Autodesk Inventor part; units mm, degrees
(part 3 of 16)
  spline S11 degree 3 poles (-7.8004, 116.1965) (-7.729, 116.082) (-7.6593, 115.9666) (-7.5915, 115.85) (-7.5548, 115.787) (-7.5187, 115.7236) (-7.4832, 115.66) (-7.4495, 115.5997) (-7.4164, 115.5392) (-7.3838, 115.4783) (-7.3531, 115.4209) (-7.3228, 115.3632) (-7.2931, 115.3052) (-7.2652, 115.2507) (-7.2377, 115.196) (-7.2107, 115.141) (-7.1855, 115.0895) (-7.1607, 115.0378) (-7.1363, 114.9858) (-7.1136, 114.9374) (-7.0914, 114.8888) (-7.0695, 114.8399) (-7.0493, 114.7947) (-7.0295, 114.7492) (-7.01, 114.7036) (-6.9921, 114.6615) (-6.9746, 114.6193) (-6.9574, 114.577) (-6.9417, 114.5382) (-6.9264, 114.4993) (-6.9114, 114.4603) (-6.8977, 114.4249) (-6.8844, 114.3893) (-6.8714, 114.3537) (-6.8598, 114.3217) (-6.8484, 114.2896) (-6.8373, 114.2574) (-6.8227, 114.2149) (-6.8087, 114.1721) (-6.7951, 114.1292) (-6.792, 114.1196) (-6.789, 114.11) (-6.7858, 114.1005) (-6.7828, 114.0911) (-6.7796, 114.0818) (-6.7764, 114.0725) (-6.7732, 114.0634) (-6.7699, 114.0544) (-6.7666, 114.0453) (-6.7633, 114.0365) (-6.76, 114.0277) (-6.7566, 114.0189) (-6.7532, 114.0102) (-6.7497, 114.0016) (-6.7462, 113.9931) (-6.7427, 113.9847) (-6.7391, 113.9763) (-6.7355, 113.9679) (-6.7318, 113.9597) (-6.7281, 113.9515) (-6.7243, 113.9433) (-6.7205, 113.9352) (-6.7166, 113.9272) (-6.7127, 113.9192) (-6.7087, 113.9113) (-6.7046, 113.9034) (-6.7004, 113.8955) (-6.6962, 113.8877) (-6.6919, 113.8799) (-6.6875, 113.8722) (-6.683, 113.8644) (-6.6784, 113.8566) (-6.6737, 113.849) (-6.6689, 113.8412) (-6.6639, 113.8335) (-6.6588, 113.8259) (-6.6536, 113.8181) (-6.6482, 113.8104) (-6.6426, 113.8028) (-6.6368, 113.7949) (-6.6309, 113.7871) (-6.6247, 113.7795) (-6.6182, 113.7715) (-6.6115, 113.7636) (-6.6046, 113.7559) (-6.5972, 113.7476) (-6.5896, 113.7396) (-6.5817, 113.7318) (-6.5731, 113.7234) (-6.5643, 113.7152) (-6.5551, 113.7074) (-6.5451, 113.6988) (-6.5346, 113.6906) (-6.5239, 113.6828) (-6.5119, 113.6741) (-6.4995, 113.666) (-6.4867, 113.6585) (-6.4723, 113.65) (-6.4575, 113.6424) (-6.4423, 113.6356) (-6.4252, 113.628) (-6.4076, 113.6214) (-6.3897, 113.6161) (-6.3697, 113.6101) (-6.3494, 113.6056) (-6.3288, 113.6026) (-6.3064, 113.5994) (-6.2838, 113.5978) (-6.2613, 113.5983) (-6.2398, 113.5988) (-6.2183, 113.6012) (-6.1969, 113.6039) (-6.0912, 113.6175) (-5.987, 113.6399) (-5.8819, 113.6571) (-5.7768, 113.6744) (-5.6709, 113.6865) (-5.5664, 113.7076) (-5.5453, 113.7118) (-5.5242, 113.7165) (-5.5036, 113.7229) (-5.4821, 113.7296) (-5.4612, 113.7383) (-5.4411, 113.7486) (-5.4225, 113.758) (-5.4047, 113.7688) (-5.3877, 113.7808) (-5.3724, 113.7916) (-5.3579, 113.8034) (-5.3441, 113.8161) (-5.3319, 113.8274) (-5.3203, 113.8394) (-5.3094, 113.852) (-5.2997, 113.8632) (-5.2905, 113.8749) (-5.2819, 113.887) (-5.2742, 113.8978) (-5.267, 113.9089) (-5.2602, 113.9203) (-5.254, 113.9307) (-5.2483, 113.9412) (-5.2428, 113.952) (-5.2379, 113.9619) (-5.2332, 113.9719) (-5.2288, 113.9821) (-5.2247, 113.9916) (-5.2209, 114.0012) (-5.2174, 114.0109) (-5.214, 114.0201) (-5.2108, 114.0293) (-5.2078, 114.0387) (-5.205, 114.0477) (-5.2024, 114.0567) (-5.1999, 114.0658) (-5.1975, 114.0746) (-5.1953, 114.0835) (-5.1932, 114.0924) (-5.1912, 114.1012) (-5.1893, 114.1099) (-5.1875, 114.1188) (-5.1858, 114.1275) (-5.1842, 114.1363) (-5.1828, 114.145) (-5.1813, 114.1538) (-5.18, 114.1626) (-5.1788, 114.1714) (-5.1776, 114.1802) (-5.1765, 114.1891) (-5.1755, 114.198) (-5.1745, 114.2069) (-5.1736, 114.2159) (-5.1728, 114.2248) (-5.172, 114.2339) (-5.1713, 114.243) (-5.1707, 114.2521) (-5.17, 114.2614) (-5.1695, 114.2706) (-5.1691, 114.2799) (-5.1687, 114.2893) (-5.1683, 114.2987) (-5.168, 114.3082) (-5.1678, 114.3178) (-5.1676, 114.3274) (-5.1675, 114.337) (-5.1674, 114.3469) (-5.1674, 114.3567) (-5.1675, 114.3666) (-5.1676, 114.3766) (-5.1678, 114.3867) (-5.1679, 114.3967) (-5.1687, 114.4417) (-5.1692, 114.4867) (-5.1689, 114.5317) (-5.1688, 114.5658) (-5.1682, 114.5998) (-5.1674, 114.6339) (-5.1666, 114.6718) (-5.1653, 114.7097) (-5.1638, 114.7476) (-5.162, 114.7894) (-5.1599, 114.8311) (-5.1575, 114.8729) (-5.1548, 114.9185) (-5.1517, 114.9641) (-5.1482, 115.0097) (-5.1444, 115.0591) (-5.1401, 115.1085) (-5.1354, 115.1579) (-5.1304, 115.2112) (-5.1249, 115.2643) (-5.1189, 115.3175) (-5.1125, 115.3745) (-5.1055, 115.4314) (-5.0981, 115.4883) (-5.0901, 115.549) (-5.0816, 115.6097) (-5.0726, 115.6703) (-5.063, 115.7347) (-5.0528, 115.7991) (-5.0421, 115.8633) (-5.0307, 115.9314) (-5.0187, 115.9994) (-5.0061, 116.0672) (-4.9929, 116.1389) (-4.9789, 116.2105) (-4.9643, 116.2819) (-4.9374, 116.4141) (-4.9084, 116.5458) (-4.8774, 116.677) knots 0 0 0 0 0.057795 0.057795 0.057795 0.089038 0.089038 0.089038 0.118617 0.118617 0.118617 0.14653 0.14653 0.14653 0.172778 0.172778 0.172778 0.19736 0.19736 0.19736 0.220277 0.220277 0.220277 0.241529 0.241529 0.241529 0.261115 0.261115 0.261115 0.279036 0.279036 0.279036 0.295292 0.295292 0.295292 0.309882 0.309882 0.309882 0.329164 0.329164 0.329164 0.333477 0.333477 0.333477 0.337694 0.337694 0.337694 0.34182 0.34182 0.34182 0.345864 0.345864 0.345864 0.349834 0.349834 0.349834 0.353742 0.353742 0.353742 0.3576 0.3576 0.3576 0.361424 0.361424 0.361424 0.365232 0.365232 0.365232 0.369048 0.369048 0.369048 0.372899 0.372899 0.372899 0.376819 0.376819 0.376819 0.380853 0.380853 0.380853 0.385052 0.385052 0.385052 0.389482 0.389482 0.389482 0.394225 0.394225 0.394225 0.399381 0.399381 0.399381 0.405067 0.405067 0.405067 0.411413 0.411413 0.411413 0.418548 0.418548 0.418548 0.426565 0.426565 0.426565 0.435472 0.435472 0.435472 0.445133 0.445133 0.445133 0.45436 0.45436 0.45436 0.5 0.5 0.5 0.54564 0.54564 0.54564 0.554867 0.554867 0.554867 0.564528 0.564528 0.564528 0.573435 0.573435 0.573435 0.581452 0.581452 0.581452 0.588587 0.588587 0.588587 0.594933 0.594933 0.594933 0.600619 0.600619 0.600619 0.605775 0.605775 0.605775 0.610518 0.610518 0.610518 0.614948 0.614948 0.614948 0.619147 0.619147 0.619147 0.623181 0.623181 0.623181 0.627101 0.627101 0.627101 0.630952 0.630952 0.630952 0.634768 0.634768 0.634768 0.638576 0.638576 0.638576 0.6424 0.6424 0.6424 0.646258 0.646258 0.646258 0.650166 0.650166 0.650166 0.654136 0.654136 0.654136 0.65818 0.65818 0.65818 0.662306 0.662306 0.662306 0.666523 0.666523 0.666523 0.670836 0.670836 0.670836 0.690118 0.690118 0.690118 0.704708 0.704708 0.704708 0.720964 0.720964 0.720964 0.738885 0.738885 0.738885 0.758471 0.758471 0.758471 0.779723 0.779723 0.779723 0.80264 0.80264 0.80264 0.827222 0.827222 0.827222 0.85347 0.85347 0.85347 0.881383 0.881383 0.881383 0.910962 0.910962 0.910962 0.942205 0.942205 0.942205 1 1 1 1
  arc A213 (-7.8004, 116.1965) -> (-8.9334, 115.9487) centre (0.0435, 77.6158) ccw
  spline S12 degree 3 poles (-11.7902, 115.1652) (-11.7073, 115.0589) (-11.6259, 114.9513) (-11.5462, 114.8425) (-11.5032, 114.7836) (-11.4606, 114.7244) (-11.4186, 114.6648) (-11.3789, 114.6084) (-11.3396, 114.5516) (-11.3008, 114.4945) (-11.2643, 114.4406) (-11.2282, 114.3864) (-11.1925, 114.3319) (-11.1591, 114.2806) (-11.126, 114.229) (-11.0934, 114.1771) (-11.0629, 114.1286) (-11.0329, 114.0797) (-11.0032, 114.0306) (-10.9756, 113.9848) (-10.9484, 113.9388) (-10.9216, 113.8925) (-10.8967, 113.8496) (-10.8722, 113.8065) (-10.8481, 113.7631) (-10.8259, 113.7232) (-10.8041, 113.683) (-10.7826, 113.6427) (-10.7629, 113.6058) (-10.7436, 113.5687) (-10.7246, 113.5315) (-10.7073, 113.4977) (-10.6904, 113.4637) (-10.6737, 113.4296) (-10.6588, 113.399) (-10.6441, 113.3683) (-10.6297, 113.3375) (-10.6108, 113.2967) (-10.5924, 113.2556) (-10.5743, 113.2144) (-10.5703, 113.2052) (-10.5662, 113.1959) (-10.5621, 113.1868) (-10.5581, 113.1778) (-10.554, 113.1689) (-10.5498, 113.16) (-10.5457, 113.1512) (-10.5415, 113.1426) (-10.5372, 113.1339) (-10.5331, 113.1255) (-10.5288, 113.117) (-10.5245, 113.1087) (-10.5202, 113.1004) (-10.5159, 113.0922) (-10.5115, 113.0841) (-10.5071, 113.0761) (-10.5027, 113.0681) (-10.4982, 113.0602) (-10.4937, 113.0524) (-10.4891, 113.0446) (-10.4845, 113.0369) (-10.4799, 113.0293) (-10.4752, 113.0217) (-10.4704, 113.0141) (-10.4656, 113.0066) (-10.4607, 112.9992) (-10.4558, 112.9919) (-10.4508, 112.9845) (-10.4457, 112.9772) (-10.4404, 112.97) (-10.4352, 112.9627) (-10.4298, 112.9555) (-10.4243, 112.9484) (-10.4187, 112.9411) (-10.413, 112.934) (-10.4071, 112.927) (-10.4011, 112.9198) (-10.3949, 112.9126) (-10.3886, 112.9057) (-10.382, 112.8984) (-10.3752, 112.8913) (-10.3683, 112.8844) (-10.361, 112.877) (-10.3535, 112.8699) (-10.3459, 112.863) (-10.3377, 112.8556) (-10.3292, 112.8484) (-10.3206, 112.8415) (-10.3112, 112.834) (-10.3015, 112.8268) (-10.2916, 112.82) (-10.2807, 112.8124) (-10.2694, 112.8053) (-10.2579, 112.7987) (-10.2451, 112.7913) (-10.2319, 112.7845) (-10.2184, 112.7784) (-10.2032, 112.7715) (-10.1877, 112.7655) (-10.1719, 112.7603) (-10.1541, 112.7545) (-10.1359, 112.7499) (-10.1175, 112.7464) (-10.097, 112.7426) (-10.0763, 112.7402) (-10.0555, 112.7394) (-10.033, 112.7385) (-10.0103, 112.7393) (-9.988, 112.7422) (-9.9666, 112.7449) (-9.9455, 112.7495) (-9.9245, 112.7545) (-9.8208, 112.779) (-9.7195, 112.8122) (-9.6168, 112.8403) (-9.5141, 112.8685) (-9.41, 112.8916) (-9.3083, 112.9235) (-9.2877, 112.9299) (-9.2672, 112.9367) (-9.2475, 112.9453) (-9.2268, 112.9542) (-9.2069, 112.965) (-9.1879, 112.9773) (-9.1705, 112.9887) (-9.1539, 113.0012) (-9.1382, 113.015) (-9.1242, 113.0273) (-9.1109, 113.0406) (-9.0986, 113.0547) (-9.0876, 113.0672) (-9.0773, 113.0803) (-9.0678, 113.094) (-9.0593, 113.1061) (-9.0514, 113.1187) (-9.0441, 113.1316) (-9.0376, 113.1432) (-9.0316, 113.155) (-9.026, 113.167) (-9.021, 113.178) (-9.0163, 113.1891) (-9.0121, 113.2003) (-9.0081, 113.2107) (-9.0045, 113.2212) (-9.0013, 113.2317) (-8.9982, 113.2416) (-8.9954, 113.2516) (-8.9929, 113.2616) (-8.9904, 113.2711) (-8.9883, 113.2806) (-8.9863, 113.2902) (-8.9844, 113.2995) (-8.9827, 113.3087) (-8.9812, 113.318) (-8.9798, 113.3271) (-8.9785, 113.3361) (-8.9774, 113.3452) (-8.9763, 113.3541) (-8.9753, 113.3631) (-8.9745, 113.372) (-8.9737, 113.3809) (-8.973, 113.3898) (-8.9725, 113.3986) (-8.972, 113.4075) (-8.9716, 113.4164) (-8.9713, 113.4253) (-8.971, 113.4342) (-8.9708, 113.4431) (-8.9708, 113.452) (-8.9707, 113.461) (-8.9707, 113.47) (-8.9709, 113.479) (-8.971, 113.4882) (-8.9713, 113.4973) (-8.9716, 113.5064) (-8.972, 113.5156) (-8.9724, 113.5249) (-8.973, 113.5342) (-8.9735, 113.5436) (-8.9742, 113.553) (-8.9749, 113.5624) (-8.9756, 113.572) (-8.9765, 113.5816) (-8.9774, 113.5912) (-8.9783, 113.601) (-8.9793, 113.6108) (-8.9804, 113.6205) (-8.9816, 113.6305) (-8.9828, 113.6405) (-8.984, 113.6505) (-8.9895, 113.6952) (-8.9947, 113.7399) (-8.9992, 113.7846) (-9.0026, 113.8185) (-9.0056, 113.8524) (-9.0083, 113.8864) (-9.0114, 113.9242) (-9.0142, 113.962) (-9.0166, 113.9999) (-9.0192, 114.0416) (-9.0215, 114.0834) (-9.0234, 114.1251) (-9.0255, 114.1708) (-9.0272, 114.2165) (-9.0285, 114.2622) (-9.0299, 114.3117) (-9.0308, 114.3613) (-9.0313, 114.4109) (-9.0318, 114.4644) (-9.0319, 114.5179) (-9.0315, 114.5713) (-9.0311, 114.6287) (-9.0301, 114.6861) (-9.0287, 114.7434) (-9.0271, 114.8046) (-9.025, 114.8659) (-9.0224, 114.927) (-9.0196, 114.9921) (-9.0162, 115.0572) (-9.0122, 115.1222) (-9.008, 115.1911) (-9.0032, 115.2599) (-8.9978, 115.3287) (-8.992, 115.4014) (-8.9856, 115.4741) (-8.9786, 115.5466) (-8.9656, 115.6809) (-8.9505, 115.8149) (-8.9334, 115.9487) knots 0 0 0 0 0.057795 0.057795 0.057795 0.089038 0.089038 0.089038 0.118617 0.118617 0.118617 0.14653 0.14653 0.14653 0.172778 0.172778 0.172778 0.19736 0.19736 0.19736 0.220277 0.220277 0.220277 0.241529 0.241529 0.241529 0.261115 0.261115 0.261115 0.279036 0.279036 0.279036 0.295292 0.295292 0.295292 0.309882 0.309882 0.309882 0.329164 0.329164 0.329164 0.333477 0.333477 0.333477 0.337694 0.337694 0.337694 0.34182 0.34182 0.34182 0.345864 0.345864 0.345864 0.349834 0.349834 0.349834 0.353742 0.353742 0.353742 0.3576 0.3576 0.3576 0.361424 0.361424 0.361424 0.365232 0.365232 0.365232 0.369048 0.369048 0.369048 0.372899 0.372899 0.372899 0.376819 0.376819 0.376819 0.380853 0.380853 0.380853 0.385052 0.385052 0.385052 0.389482 0.389482 0.389482 0.394225 0.394225 0.394225 0.399381 0.399381 0.399381 0.405067 0.405067 0.405067 0.411413 0.411413 0.411413 0.418548 0.418548 0.418548 0.426565 0.426565 0.426565 0.435472 0.435472 0.435472 0.445133 0.445133 0.445133 0.45436 0.45436 0.45436 0.5 0.5 0.5 0.54564 0.54564 0.54564 0.554867 0.554867 0.554867 0.564528 0.564528 0.564528 0.573435 0.573435 0.573435 0.581452 0.581452 0.581452 0.588587 0.588587 0.588587 0.594933 0.594933 0.594933 0.600619 0.600619 0.600619 0.605775 0.605775 0.605775 0.610518 0.610518 0.610518 0.614948 0.614948 0.614948 0.619147 0.619147 0.619147 0.623181 0.623181 0.623181 0.627101 0.627101 0.627101 0.630952 0.630952 0.630952 0.634768 0.634768 0.634768 0.638576 0.638576 0.638576 0.6424 0.6424 0.6424 0.646258 0.646258 0.646258 0.650166 0.650166 0.650166 0.654136 0.654136 0.654136 0.65818 0.65818 0.65818 0.662306 0.662306 0.662306 0.666523 0.666523 0.666523 0.670836 0.670836 0.670836 0.690118 0.690118 0.690118 0.704708 0.704708 0.704708 0.720964 0.720964 0.720964 0.738885 0.738885 0.738885 0.758471 0.758471 0.758471 0.779723 0.779723 0.779723 0.80264 0.80264 0.80264 0.827222 0.827222 0.827222 0.85347 0.85347 0.85347 0.881383 0.881383 0.881383 0.910962 0.910962 0.910962 0.942205 0.942205 0.942205 1 1 1 1
  arc A214 (-11.7902, 115.1652) -> (-12.8911, 114.8003) centre (0.0435, 77.6158) ccw
  spline S13 degree 3 poles (-15.6504, 113.7226) (-15.5568, 113.6255) (-15.4646, 113.527) (-15.374, 113.4271) (-15.325, 113.3731) (-15.2765, 113.3186) (-15.2285, 113.2638) (-15.1831, 113.2118) (-15.1381, 113.1595) (-15.0936, 113.1067) (-15.0516, 113.0569) (-15.01, 113.0068) (-14.9689, 112.9563) (-14.9302, 112.9088) (-14.892, 112.8609) (-14.8541, 112.8127) (-14.8187, 112.7676) (-14.7837, 112.7222) (-14.7491, 112.6764) (-14.7168, 112.6338) (-14.6849, 112.5908) (-14.6535, 112.5476) (-14.6242, 112.5075) (-14.5954, 112.4672) (-14.5669, 112.4266) (-14.5406, 112.3892) (-14.5147, 112.3516) (-14.4891, 112.3137) (-14.4657, 112.2791) (-14.4426, 112.2442) (-14.4198, 112.2091) (-14.3991, 112.1773) (-14.3787, 112.1454) (-14.3586, 112.1132) (-14.3405, 112.0843) (-14.3227, 112.0553) (-14.3052, 112.0261) (-14.2821, 111.9875) (-14.2595, 111.9486) (-14.2372, 111.9095) (-14.2322, 111.9008) (-14.2273, 111.892) (-14.2222, 111.8833) (-14.2173, 111.8748) (-14.2122, 111.8664) (-14.2071, 111.8579) (-14.2021, 111.8497) (-14.1971, 111.8415) (-14.1919, 111.8334) (-14.1869, 111.8254) (-14.1818, 111.8175) (-14.1766, 111.8096) (-14.1715, 111.8018) (-14.1663, 111.7941) (-14.1611, 111.7865) (-14.1559, 111.779) (-14.1507, 111.7715) (-14.1454, 111.7641) (-14.1401, 111.7568) (-14.1348, 111.7496) (-14.1293, 111.7424) (-14.124, 111.7353) (-14.1185, 111.7282) (-14.1129, 111.7212) (-14.1074, 111.7143) (-14.1018, 111.7074) (-14.096, 111.7006) (-14.0903, 111.6938) (-14.0845, 111.6871) (-14.0785, 111.6804) (-14.0725, 111.6737) (-14.0664, 111.6671) (-14.0602, 111.6606) (-14.0539, 111.654) (-14.0475, 111.6475) (-14.0409, 111.6412) (-14.0341, 111.6346) (-14.0273, 111.6282) (-14.0202, 111.6219) (-14.0129, 111.6154) (-14.0055, 111.609) (-13.9979, 111.6028) (-13.9898, 111.5963) (-13.9817, 111.59) (-13.9733, 111.5839) (-13.9643, 111.5774) (-13.9552, 111.5711) (-13.9459, 111.5652) (-13.9357, 111.5587) (-13.9254, 111.5526) (-13.9148, 111.5468) (-13.9032, 111.5404) (-13.8913, 111.5346) (-13.8791, 111.5292) (-13.8656, 111.5232) (-13.8517, 111.5178) (-13.8377, 111.5131) (-13.8219, 111.5079) (-13.8058, 111.5035) (-13.7895, 111.5) (-13.7712, 111.4961) (-13.7526, 111.4934) (-13.734, 111.4918) (-13.7132, 111.4902) (-13.6924, 111.49) (-13.6716, 111.4914) (-13.6491, 111.4928) (-13.6266, 111.496) (-13.6047, 111.5012) (-13.5838, 111.5061) (-13.5633, 111.5129) (-13.5429, 111.52) (-13.4423, 111.5553) (-13.345, 111.5989) (-13.2458, 111.6376) (-13.1467, 111.6763) (-13.0456, 111.7102) (-12.9477, 111.7525) (-12.9279, 111.7611) (-12.9083, 111.77) (-12.8895, 111.7805) (-12.8699, 111.7916) (-12.8512, 111.8045) (-12.8337, 111.8187) (-12.8175, 111.8318) (-12.8023, 111.846) (-12.7882, 111.8613) (-12.7755, 111.8751) (-12.7637, 111.8897) (-12.7529, 111.9049) (-12.7432, 111.9185) (-12.7344, 111.9327) (-12.7263, 111.9473) (-12.7192, 111.9602) (-12.7126, 111.9735) (-12.7067, 111.9871) (-12.7015, 111.9993) (-12.6967, 112.0117) (-12.6924, 112.0243) (-12.6886, 112.0357) (-12.6851, 112.0472) (-12.682, 112.0588) (-12.6792, 112.0695) (-12.6768, 112.0803) (-12.6746, 112.0912) (-12.6726, 112.1013) (-12.6708, 112.1115) (-12.6694, 112.1218) (-12.668, 112.1315) (-12.6668, 112.1412) (-12.6658, 112.1509) (-12.6649, 112.1603) (-12.6642, 112.1697) (-12.6637, 112.1791) (-12.6632, 112.1882) (-12.6629, 112.1974) (-12.6627, 112.2065) (-12.6625, 112.2155) (-12.6625, 112.2245) (-12.6626, 112.2335) (-12.6628, 112.2424) (-12.663, 112.2513) (-12.6634, 112.2602) (-12.6638, 112.2691) (-12.6644, 112.2779) (-12.665, 112.2868) (-12.6656, 112.2957) (-12.6664, 112.3046) (-12.6673, 112.3135) (-12.6682, 112.3224) (-12.6691, 112.3314) (-12.6702, 112.3403) (-12.6713, 112.3494) (-12.6725, 112.3584) (-12.6738, 112.3674) (-12.6752, 112.3766) (-12.6766, 112.3858) (-12.6781, 112.3949) (-12.6796, 112.4042) (-12.6812, 112.4135) (-12.6829, 112.4228) (-12.6847, 112.4323) (-12.6865, 112.4417) (-12.6884, 112.4512) (-12.6904, 112.4608) (-12.6924, 112.4704) (-12.6945, 112.48) (-12.6967, 112.4899) (-12.699, 112.4997) (-12.7012, 112.5095) (-12.7114, 112.5533) (-12.7211, 112.5972) (-12.7303, 112.6413) (-12.7372, 112.6746) (-12.7438, 112.708) (-12.7501, 112.7415) (-12.7571, 112.7788) (-12.7638, 112.8161) (-12.7701, 112.8535) (-12.7771, 112.8947) (-12.7837, 112.936) (-12.79, 112.9774) (-12.7969, 113.0226) (-12.8033, 113.0678) (-12.8094, 113.1131) (-12.8159, 113.1623) (-12.822, 113.2115) (-12.8277, 113.2608) (-12.8339, 113.3139) (-12.8395, 113.3671) (-12.8447, 113.4203) (-12.8503, 113.4774) (-12.8553, 113.5345) (-12.8599, 113.5917) (-12.8647, 113.6528) (-12.869, 113.7139) (-12.8728, 113.775) (-12.8768, 113.84) (-12.8802, 113.9051) (-12.8831, 113.9701) (-12.8861, 114.0391) (-12.8885, 114.1081) (-12.8903, 114.1771) (-12.8922, 114.25) (-12.8934, 114.3229) (-12.8941, 114.3958) (-12.8952, 114.5306) (-12.8941, 114.6655) (-12.8911, 114.8003) knots 0 0 0 0 0.057795 0.057795 0.057795 0.089038 0.089038 0.089038 0.118617 0.118617 0.118617 0.14653 0.14653 0.14653 0.172778 0.172778 0.172778 0.19736 0.19736 0.19736 0.220277 0.220277 0.220277 0.241529 0.241529 0.241529 0.261115 0.261115 0.261115 0.279036 0.279036 0.279036 0.295292 0.295292 0.295292 0.309882 0.309882 0.309882 0.329164 0.329164 0.329164 0.333477 0.333477 0.333477 0.337694 0.337694 0.337694 0.34182 0.34182 0.34182 0.345864 0.345864 0.345864 0.349834 0.349834 0.349834 0.353742 0.353742 0.353742 0.3576 0.3576 0.3576 0.361424 0.361424 0.361424 0.365232 0.365232 0.365232 0.369048 0.369048 0.369048 0.372899 0.372899 0.372899 0.376819 0.376819 0.376819 0.380853 0.380853 0.380853 0.385052 0.385052 0.385052 0.389482 0.389482 0.389482 0.394225 0.394225 0.394225 0.399381 0.399381 0.399381 0.405067 0.405067 0.405067 0.411413 0.411413 0.411413 0.418548 0.418548 0.418548 0.426565 0.426565 0.426565 0.435472 0.435472 0.435472 0.445133 0.445133 0.445133 0.45436 0.45436 0.45436 0.5 0.5 0.5 0.54564 0.54564 0.54564 0.554867 0.554867 0.554867 0.564528 0.564528 0.564528 0.573435 0.573435 0.573435 0.581452 0.581452 0.581452 0.588587 0.588587 0.588587 0.594933 0.594933 0.594933 0.600619 0.600619 0.600619 0.605775 0.605775 0.605775 0.610518 0.610518 0.610518 0.614948 0.614948 0.614948 0.619147 0.619147 0.619147 0.623181 0.623181 0.623181 0.627101 0.627101 0.627101 0.630952 0.630952 0.630952 0.634768 0.634768 0.634768 0.638576 0.638576 0.638576 0.6424 0.6424 0.6424 0.646258 0.646258 0.646258 0.650166 0.650166 0.650166 0.654136 0.654136 0.654136 0.65818 0.65818 0.65818 0.662306 0.662306 0.662306 0.666523 0.666523 0.666523 0.670836 0.670836 0.670836 0.690118 0.690118 0.690118 0.704708 0.704708 0.704708 0.720964 0.720964 0.720964 0.738885 0.738885 0.738885 0.758471 0.758471 0.758471 0.779723 0.779723 0.779723 0.80264 0.80264 0.80264 0.827222 0.827222 0.827222 0.85347 0.85347 0.85347 0.881383 0.881383 0.881383 0.910962 0.910962 0.910962 0.942205 0.942205 0.942205 1 1 1 1
  arc A215 (-15.6504, 113.7226) -> (-16.7071, 113.2446) centre (0.0435, 77.6158) ccw
  spline S14 degree 3 poles (-19.3386, 111.8843) (-19.2353, 111.7975) (-19.1334, 111.7092) (-19.0328, 111.6193) (-18.9785, 111.5707) (-18.9246, 111.5217) (-18.8711, 111.4721) (-18.8205, 111.4252) (-18.7702, 111.3778) (-18.7205, 111.33) (-18.6735, 111.2849) (-18.6269, 111.2394) (-18.5807, 111.1934) (-18.5373, 111.1502) (-18.4943, 111.1067) (-18.4516, 111.0627) (-18.4117, 111.0215) (-18.3721, 110.98) (-18.3329, 110.9381) (-18.2964, 110.8991) (-18.2602, 110.8597) (-18.2243, 110.82) (-18.1911, 110.7832) (-18.1582, 110.7461) (-18.1256, 110.7087) (-18.0955, 110.6743) (-18.0658, 110.6395) (-18.0364, 110.6046) (-18.0095, 110.5725) (-17.9829, 110.5403) (-17.9565, 110.5078) (-17.9326, 110.4783) (-17.909, 110.4487) (-17.8857, 110.4188) (-17.8647, 110.392) (-17.8439, 110.365) (-17.8235, 110.3378) (-17.7964, 110.3018) (-17.7699, 110.2655) (-17.7437, 110.2289) (-17.7378, 110.2207) (-17.7319, 110.2125) (-17.726, 110.2044) (-17.7202, 110.1965) (-17.7143, 110.1886) (-17.7083, 110.1808) (-17.7025, 110.1731) (-17.6966, 110.1655) (-17.6907, 110.1579) (-17.6848, 110.1505) (-17.6789, 110.1431) (-17.6729, 110.1358) (-17.667, 110.1287) (-17.6611, 110.1216) (-17.6551, 110.1145) (-17.6492, 110.1076) (-17.6432, 110.1007) (-17.6371, 110.0939) (-17.6311, 110.0872) (-17.625, 110.0805) (-17.6189, 110.074) (-17.6128, 110.0674) (-17.6066, 110.061) (-17.6004, 110.0546) (-17.5941, 110.0483) (-17.5878, 110.0421) (-17.5814, 110.0359) (-17.575, 110.0297) (-17.5685, 110.0236) (-17.5619, 110.0177) (-17.5552, 110.0116) (-17.5485, 110.0057) (-17.5416, 109.9999) (-17.5346, 109.994) (-17.5276, 109.9882) (-17.5204, 109.9825) (-17.513, 109.9767) (-17.5054, 109.9711) (-17.4978, 109.9656) (-17.4898, 109.9598) (-17.4818, 109.9543) (-17.4736, 109.9489) (-17.4649, 109.9433) (-17.4561, 109.9379) (-17.4471, 109.9327) (-17.4376, 109.9271) (-17.4278, 109.9219) (-17.4179, 109.9169) (-17.4072, 109.9115) (-17.3962, 109.9065) (-17.3851, 109.9019) (-17.3729, 109.8968) (-17.3604, 109.8922) (-17.3478, 109.8881) (-17.3337, 109.8835) (-17.3194, 109.8797) (-17.3049, 109.8765) (-17.2886, 109.8729) (-17.2722, 109.8702) (-17.2556, 109.8684) (-17.237, 109.8665) (-17.2182, 109.8657) (-17.1995, 109.8661) (-17.1787, 109.8666) (-17.158, 109.8687) (-17.1375, 109.8722) (-17.1152, 109.876) (-17.0932, 109.8815) (-17.0719, 109.8889) (-17.0516, 109.896) (-17.032, 109.9049) (-17.0125, 109.9141) (-16.9161, 109.9597) (-16.8239, 110.0132) (-16.7293, 110.0621) (-16.6347, 110.111) (-16.5377, 110.1553) (-16.4448, 110.2076) (-16.426, 110.2182) (-16.4074, 110.2291) (-16.3899, 110.2415) (-16.3715, 110.2546) (-16.3543, 110.2693) (-16.3383, 110.2853) (-16.3236, 110.3) (-16.3099, 110.3158) (-16.2975, 110.3324) (-16.2863, 110.3474) (-16.2761, 110.3632) (-16.2669, 110.3795) (-16.2588, 110.394) (-16.2515, 110.409) (-16.245, 110.4244) (-16.2392, 110.438) (-16.2341, 110.4519) (-16.2297, 110.4661) (-16.2257, 110.4787) (-16.2223, 110.4916) (-16.2193, 110.5045) (-16.2167, 110.5162) (-16.2144, 110.5281) (-16.2126, 110.54) (-16.2109, 110.5509) (-16.2096, 110.5619) (-16.2086, 110.5729) (-16.2076, 110.5832) (-16.207, 110.5936) (-16.2066, 110.6039) (-16.2062, 110.6137) (-16.206, 110.6235) (-16.2061, 110.6333) (-16.2062, 110.6427) (-16.2065, 110.6521) (-16.2069, 110.6615) (-16.2074, 110.6706) (-16.208, 110.6798) (-16.2088, 110.6889) (-16.2096, 110.6978) (-16.2105, 110.7068) (-16.2116, 110.7157) (-16.2126, 110.7245) (-16.2138, 110.7334) (-16.2152, 110.7422) (-16.2165, 110.751) (-16.2179, 110.7597) (-16.2195, 110.7685) (-16.2211, 110.7773) (-16.2228, 110.786) (-16.2245, 110.7948) (-16.2264, 110.8036) (-16.2283, 110.8124) (-16.2303, 110.8212) (-16.2323, 110.83) (-16.2345, 110.8389) (-16.2367, 110.8477) (-16.239, 110.8567) (-16.2413, 110.8657) (-16.2438, 110.8746) (-16.2463, 110.8837) (-16.2489, 110.8928) (-16.2515, 110.9018) (-16.2543, 110.9111) (-16.2571, 110.9203) (-16.26, 110.9295) (-16.2629, 110.9389) (-16.2659, 110.9482) (-16.2691, 110.9576) (-16.2722, 110.9671) (-16.2755, 110.9766) (-16.2788, 110.9861) (-16.2935, 111.0287) (-16.3078, 111.0713) (-16.3215, 111.1142) (-16.3318, 111.1466) (-16.3419, 111.1792) (-16.3516, 111.2118) (-16.3625, 111.2481) (-16.373, 111.2846) (-16.3833, 111.3211) (-16.3945, 111.3614) (-16.4054, 111.4017) (-16.416, 111.4422) (-16.4275, 111.4864) (-16.4387, 111.5308) (-16.4494, 111.5752) (-16.4611, 111.6234) (-16.4723, 111.6717) (-16.4831, 111.7201) (-16.4948, 111.7723) (-16.506, 111.8246) (-16.5167, 111.877) (-16.5282, 111.9332) (-16.5392, 111.9895) (-16.5497, 112.0459) (-16.5609, 112.1061) (-16.5716, 112.1664) (-16.5817, 112.2268) (-16.5925, 112.291) (-16.6027, 112.3554) (-16.6123, 112.4198) (-16.6226, 112.4881) (-16.6321, 112.5564) (-16.6412, 112.6248) (-16.6507, 112.6971) (-16.6595, 112.7695) (-16.6677, 112.8419) (-16.683, 112.976) (-16.696, 113.1102) (-16.7071, 113.2446) knots 0 0 0 0 0.057795 0.057795 0.057795 0.089038 0.089038 0.089038 0.118617 0.118617 0.118617 0.14653 0.14653 0.14653 0.172778 0.172778 0.172778 0.19736 0.19736 0.19736 0.220277 0.220277 0.220277 0.241529 0.241529 0.241529 0.261115 0.261115 0.261115 0.279036 0.279036 0.279036 0.295292 0.295292 0.295292 0.309882 0.309882 0.309882 0.329164 0.329164 0.329164 0.333477 0.333477 0.333477 0.337694 0.337694 0.337694 0.34182 0.34182 0.34182 0.345864 0.345864 0.345864 0.349834 0.349834 0.349834 0.353742 0.353742 0.353742 0.3576 0.3576 0.3576 0.361424 0.361424 0.361424 0.365232 0.365232 0.365232 0.369048 0.369048 0.369048 0.372899 0.372899 0.372899 0.376819 0.376819 0.376819 0.380853 0.380853 0.380853 0.385052 0.385052 0.385052 0.389482 0.389482 0.389482 0.394225 0.394225 0.394225 0.399381 0.399381 0.399381 0.405067 0.405067 0.405067 0.411413 0.411413 0.411413 0.418548 0.418548 0.418548 0.426565 0.426565 0.426565 0.435472 0.435472 0.435472 0.445133 0.445133 0.445133 0.45436 0.45436 0.45436 0.5 0.5 0.5 0.54564 0.54564 0.54564 0.554867 0.554867 0.554867 0.564528 0.564528 0.564528 0.573435 0.573435 0.573435 0.581452 0.581452 0.581452 0.588587 0.588587 0.588587 0.594933 0.594933 0.594933 0.600619 0.600619 0.600619 0.605775 0.605775 0.605775 0.610518 0.610518 0.610518 0.614948 0.614948 0.614948 0.619147 0.619147 0.619147 0.623181 0.623181 0.623181 0.627101 0.627101 0.627101 0.630952 0.630952 0.630952 0.634768 0.634768 0.634768 0.638576 0.638576 0.638576 0.6424 0.6424 0.6424 0.646258 0.646258 0.646258 0.650166 0.650166 0.650166 0.654136 0.654136 0.654136 0.65818 0.65818 0.65818 0.662306 0.662306 0.662306 0.666523 0.666523 0.666523 0.670836 0.670836 0.670836 0.690118 0.690118 0.690118 0.704708 0.704708 0.704708 0.720964 0.720964 0.720964 0.738885 0.738885 0.738885 0.758471 0.758471 0.758471 0.779723 0.779723 0.779723 0.80264 0.80264 0.80264 0.827222 0.827222 0.827222 0.85347 0.85347 0.85347 0.881383 0.881383 0.881383 0.910962 0.910962 0.910962 0.942205 0.942205 0.942205 1 1 1 1
  arc A216 (-19.3386, 111.8843) -> (-20.3396, 111.2985) centre (0.0435, 77.6158) ccw
  spline S15 degree 3 poles (-22.8144, 109.6706) (-22.7027, 109.5951) (-22.5921, 109.5179) (-22.4827, 109.439) (-22.4235, 109.3964) (-22.3648, 109.3532) (-22.3064, 109.3095) (-22.2512, 109.2682) (-22.1963, 109.2263) (-22.1418, 109.184) (-22.0903, 109.144) (-22.0392, 109.1036) (-21.9885, 109.0627) (-21.9408, 109.0243) (-21.8935, 108.9855) (-21.8465, 108.9462) (-21.8024, 108.9094) (-21.7587, 108.8723) (-21.7154, 108.8347) (-21.6749, 108.7997) (-21.6348, 108.7643) (-21.595, 108.7286) (-21.5581, 108.6955) (-21.5215, 108.662) (-21.4852, 108.6282) (-21.4517, 108.5971) (-21.4185, 108.5657) (-21.3856, 108.534) (-21.3555, 108.5049) (-21.3257, 108.4757) (-21.2961, 108.4461) (-21.2692, 108.4193) (-21.2426, 108.3923) (-21.2163, 108.365) (-21.1926, 108.3405) (-21.1692, 108.3158) (-21.146, 108.2909) (-21.1153, 108.258) (-21.0851, 108.2246) (-21.0552, 108.191) (-21.0485, 108.1835) (-21.0418, 108.1759) (-21.0351, 108.1685) (-21.0285, 108.1612) (-21.0218, 108.154) (-21.015, 108.1468) (-21.0085, 108.1398) (-21.0018, 108.1328) (-20.9951, 108.1259) (-20.9885, 108.1192) (-20.9819, 108.1125) (-20.9751, 108.1058) (-20.9686, 108.0993) (-20.9619, 108.0929) (-20.9552, 108.0865) (-20.9486, 108.0802) (-20.9419, 108.074) (-20.9351, 108.0679) (-20.9285, 108.0618) (-20.9217, 108.0558) (-20.9149, 108.0499) (-20.9082, 108.0441) (-20.9014, 108.0383) (-20.8945, 108.0327) (-20.8876, 108.027) (-20.8807, 108.0214) (-20.8737, 108.016) (-20.8667, 108.0105) (-20.8596, 108.0051) (-20.8524, 107.9999) (-20.8451, 107.9946) (-20.8378, 107.9894) (-20.8304, 107.9843) (-20.8228, 107.9792) (-20.8151, 107.9742) (-20.8074, 107.9693) (-20.7994, 107.9643) (-20.7913, 107.9595) (-20.7832, 107.9548) (-20.7747, 107.9499) (-20.7661, 107.9452) (-20.7573, 107.9408) (-20.7481, 107.9361) (-20.7388, 107.9316) (-20.7294, 107.9274) (-20.7193, 107.9229) (-20.709, 107.9186) (-20.6987, 107.9147) (-20.6874, 107.9105) (-20.676, 107.9067) (-20.6644, 107.9032) (-20.6517, 107.8994) (-20.6389, 107.8962) (-20.6259, 107.8934) (-20.6114, 107.8904) (-20.5967, 107.888) (-20.582, 107.8863) (-20.5655, 107.8845) (-20.5488, 107.8835) (-20.5321, 107.8835) (-20.5134, 107.8835) (-20.4947, 107.8847) (-20.4761, 107.8871) (-20.4555, 107.8898) (-20.4351, 107.8939) (-20.415, 107.8996) (-20.3933, 107.9057) (-20.372, 107.9134) (-20.3516, 107.9231) (-20.3322, 107.9323) (-20.3135, 107.9432) (-20.2951, 107.9544) (-20.204, 108.0098) (-20.1179, 108.0726) (-20.029, 108.1311) (-19.94, 108.1896) (-19.8482, 108.2438) (-19.7613, 108.3055) (-19.7437, 108.318) (-19.7263, 108.3308) (-19.7102, 108.345) (-19.6932, 108.3599) (-19.6777, 108.3764) (-19.6634, 108.3939) (-19.6503, 108.4101) (-19.6384, 108.4272) (-19.6278, 108.4451) (-19.6182, 108.4612) (-19.6097, 108.4779) (-19.6023, 108.4951) (-19.5958, 108.5104) (-19.59, 108.5261) (-19.5852, 108.542) (-19.5809, 108.5562) (-19.5773, 108.5706) (-19.5743, 108.5851) (-19.5717, 108.5981) (-19.5696, 108.6112) (-19.5681, 108.6244) (-19.5666, 108.6364) (-19.5657, 108.6484) (-19.5651, 108.6604) (-19.5646, 108.6714) (-19.5644, 108.6825) (-19.5645, 108.6936) (-19.5647, 108.7039) (-19.5651, 108.7143) (-19.5657, 108.7246) (-19.5664, 108.7344) (-19.5673, 108.7441) (-19.5684, 108.7539) (-19.5694, 108.7632) (-19.5707, 108.7725) (-19.5721, 108.7818) (-19.5735, 108.7909) (-19.5751, 108.7999) (-19.5768, 108.8089) (-19.5785, 108.8177) (-19.5804, 108.8265) (-19.5824, 108.8353) (-19.5844, 108.8439) (-19.5865, 108.8526) (-19.5887, 108.8612) (-19.591, 108.8698) (-19.5933, 108.8784) (-19.5958, 108.8869) (-19.5983, 108.8955) (-19.6009, 108.904) (-19.6036, 108.9125) (-19.6063, 108.9211) (-19.6091, 108.9297) (-19.612, 108.9382) (-19.615, 108.9468) (-19.6181, 108.9554) (-19.6212, 108.964) (-19.6244, 108.9726) (-19.6277, 108.9813) (-19.6311, 108.9899) (-19.6345, 108.9987) (-19.638, 109.0075) (-19.6416, 109.0162) (-19.6453, 109.0251) (-19.6491, 109.034) (-19.6529, 109.0428) (-19.6568, 109.0518) (-19.6608, 109.0608) (-19.6649, 109.0698) (-19.669, 109.0789) (-19.6733, 109.0881) (-19.6776, 109.0972) (-19.6966, 109.138) (-19.7153, 109.1789) (-19.7334, 109.2201) (-19.7471, 109.2513) (-19.7604, 109.2826) (-19.7735, 109.314) (-19.7882, 109.349) (-19.8024, 109.3841) (-19.8164, 109.4194) (-19.8319, 109.4583) (-19.8469, 109.4973) (-19.8617, 109.5364) (-19.8778, 109.5792) (-19.8935, 109.6221) (-19.9088, 109.6652) (-19.9254, 109.7119) (-19.9417, 109.7588) (-19.9575, 109.8058) (-19.9745, 109.8565) (-19.9911, 109.9073) (-20.0072, 109.9583) (-20.0246, 110.013) (-20.0414, 110.0678) (-20.0577, 110.1228) (-20.0752, 110.1815) (-20.0921, 110.2404) (-20.1085, 110.2994) (-20.1259, 110.3622) (-20.1428, 110.4251) (-20.1591, 110.4881) (-20.1764, 110.5549) (-20.1931, 110.6219) (-20.2092, 110.689) (-20.2262, 110.7599) (-20.2426, 110.831) (-20.2583, 110.9022) (-20.2875, 111.0339) (-20.3145, 111.166) (-20.3396, 111.2985) knots 0 0 0 0 0.057795 0.057795 0.057795 0.089038 0.089038 0.089038 0.118617 0.118617 0.118617 0.14653 0.14653 0.14653 0.172778 0.172778 0.172778 0.19736 0.19736 0.19736 0.220277 0.220277 0.220277 0.241529 0.241529 0.241529 0.261115 0.261115 0.261115 0.279036 0.279036 0.279036 0.295292 0.295292 0.295292 0.309882 0.309882 0.309882 0.329164 0.329164 0.329164 0.333477 0.333477 0.333477 0.337694 0.337694 0.337694 0.34182 0.34182 0.34182 0.345864 0.345864 0.345864 0.349834 0.349834 0.349834 0.353742 0.353742 0.353742 0.3576 0.3576 0.3576 0.361424 0.361424 0.361424 0.365232 0.365232 0.365232 0.369048 0.369048 0.369048 0.372899 0.372899 0.372899 0.376819 0.376819 0.376819 0.380853 0.380853 0.380853 0.385052 0.385052 0.385052 0.389482 0.389482 0.389482 0.394225 0.394225 0.394225 0.399381 0.399381 0.399381 0.405067 0.405067 0.405067 0.411413 0.411413 0.411413 0.418548 0.418548 0.418548 0.426565 0.426565 0.426565 0.435472 0.435472 0.435472 0.445133 0.445133 0.445133 0.45436 0.45436 0.45436 0.5 0.5 0.5 0.54564 0.54564 0.54564 0.554867 0.554867 0.554867 0.564528 0.564528 0.564528 0.573435 0.573435 0.573435 0.581452 0.581452 0.581452 0.588587 0.588587 0.588587 0.594933 0.594933 0.594933 0.600619 0.600619 0.600619 0.605775 0.605775 0.605775 0.610518 0.610518 0.610518 0.614948 0.614948 0.614948 0.619147 0.619147 0.619147 0.623181 0.623181 0.623181 0.627101 0.627101 0.627101 0.630952 0.630952 0.630952 0.634768 0.634768 0.634768 0.638576 0.638576 0.638576 0.6424 0.6424 0.6424 0.646258 0.646258 0.646258 0.650166 0.650166 0.650166 0.654136 0.654136 0.654136 0.65818 0.65818 0.65818 0.662306 0.662306 0.662306 0.666523 0.666523 0.666523 0.670836 0.670836 0.670836 0.690118 0.690118 0.690118 0.704708 0.704708 0.704708 0.720964 0.720964 0.720964 0.738885 0.738885 0.738885 0.758471 0.758471 0.758471 0.779723 0.779723 0.779723 0.80264 0.80264 0.80264 0.827222 0.827222 0.827222 0.85347 0.85347 0.85347 0.881383 0.881383 0.881383 0.910962 0.910962 0.910962 0.942205 0.942205 0.942205 1 1 1 1
  arc A217 (-22.8144, 109.6706) -> (-23.7487, 108.9834) centre (0.0435, 77.6158) ccw
  spline S16 degree 3 poles (-26.0399, 107.1057) (-25.9208, 107.0423) (-25.8027, 106.9771) (-25.6857, 106.9101) (-25.6224, 106.8738) (-25.5595, 106.8371) (-25.4969, 106.7997) (-25.4376, 106.7643) (-25.3786, 106.7285) (-25.32, 106.692) (-25.2647, 106.6577) (-25.2096, 106.6228) (-25.1549, 106.5875) (-25.1035, 106.5543) (-25.0523, 106.5206) (-25.0015, 106.4864) (-24.9538, 106.4545) (-24.9065, 106.4221) (-24.8594, 106.3893) (-24.8156, 106.3587) (-24.772, 106.3277) (-24.7287, 106.2963) (-24.6885, 106.2672) (-24.6486, 106.2378) (-24.6089, 106.208) (-24.5724, 106.1805) (-24.5361, 106.1528) (-24.5001, 106.1246) (-24.4671, 106.0989) (-24.4343, 106.0729) (-24.4018, 106.0466) (-24.3723, 106.0228) (-24.3431, 105.9987) (-24.314, 105.9743) (-24.2879, 105.9524) (-24.262, 105.9303) (-24.2363, 105.908) (-24.2024, 105.8784) (-24.1689, 105.8484) (-24.1356, 105.8181) (-24.1282, 105.8113) (-24.1207, 105.8045) (-24.1132, 105.7978) (-24.1059, 105.7912) (-24.0985, 105.7848) (-24.091, 105.7783) (-24.0838, 105.772) (-24.0764, 105.7658) (-24.069, 105.7597) (-24.0618, 105.7536) (-24.0544, 105.7477) (-24.0471, 105.7418) (-24.0398, 105.736) (-24.0326, 105.7303) (-24.0252, 105.7246) (-24.018, 105.7191) (-24.0107, 105.7136) (-24.0033, 105.7082) (-23.9961, 105.7029) (-23.9887, 105.6976) (-23.9814, 105.6925) (-23.9741, 105.6874) (-23.9667, 105.6823) (-23.9592, 105.6774) (-23.9518, 105.6725) (-23.9443, 105.6677) (-23.9368, 105.663) (-23.9292, 105.6583) (-23.9216, 105.6537) (-23.9139, 105.6492) (-23.9061, 105.6447) (-23.8983, 105.6403) (-23.8904, 105.6361) (-23.8823, 105.6317) (-23.8742, 105.6276) (-23.866, 105.6235) (-23.8575, 105.6194) (-23.849, 105.6154) (-23.8404, 105.6116) (-23.8314, 105.6076) (-23.8224, 105.6039) (-23.8132, 105.6004) (-23.8036, 105.5966) (-23.7938, 105.5932) (-23.784, 105.59) (-23.7735, 105.5865) (-23.7628, 105.5834) (-23.7521, 105.5806) (-23.7405, 105.5776) (-23.7287, 105.5749) (-23.7169, 105.5727) (-23.7039, 105.5703) (-23.6907, 105.5684) (-23.6775, 105.567) (-23.6628, 105.5655) (-23.648, 105.5647) (-23.6332, 105.5646) (-23.6165, 105.5644) (-23.5998, 105.5652) (-23.5833, 105.567) (-23.5647, 105.5689) (-23.5462, 105.572) (-23.5279, 105.5764) (-23.5077, 105.5812) (-23.4878, 105.5875) (-23.4685, 105.5952) (-23.4475, 105.6035) (-23.4271, 105.6135) (-23.4079, 105.6252) (-23.3895, 105.6364) (-23.3721, 105.6492) (-23.355, 105.6622) (-23.2701, 105.7268) (-23.1911, 105.7983) (-23.1087, 105.8658) (-23.0264, 105.9333) (-22.9407, 105.9968) (-22.8607, 106.0673) (-22.8446, 106.0815) (-22.8286, 106.096) (-22.814, 106.1119) (-22.7988, 106.1285) (-22.785, 106.1465) (-22.7727, 106.1654) (-22.7613, 106.1829) (-22.7513, 106.2011) (-22.7426, 106.22) (-22.7348, 106.237) (-22.7281, 106.2545) (-22.7225, 106.2724) (-22.7175, 106.2883) (-22.7135, 106.3045) (-22.7103, 106.3209) (-22.7075, 106.3354) (-22.7054, 106.3501) (-22.704, 106.3648) (-22.7028, 106.378) (-22.7021, 106.3913) (-22.7019, 106.4046) (-22.7017, 106.4166) (-22.702, 106.4287) (-22.7027, 106.4407) (-22.7033, 106.4517) (-22.7043, 106.4628) (-22.7056, 106.4737) (-22.7068, 106.484) (-22.7083, 106.4942) (-22.7101, 106.5044) (-22.7117, 106.5141) (-22.7136, 106.5237) (-22.7158, 106.5333) (-22.7178, 106.5425) (-22.72, 106.5516) (-22.7224, 106.5607) (-22.7248, 106.5696) (-22.7273, 106.5784) (-22.7299, 106.5871) (-22.7325, 106.5957) (-22.7353, 106.6043) (-22.7382, 106.6128) (-22.7411, 106.6212) (-22.7441, 106.6296) (-22.7472, 106.6379) (-22.7503, 106.6462) (-22.7536, 106.6545) (-22.7569, 106.6627) (-22.7603, 106.671) (-22.7638, 106.6792) (-22.7673, 106.6874) (-22.771, 106.6957) (-22.7747, 106.7039) (-22.7785, 106.712) (-22.7823, 106.7203) (-22.7862, 106.7285) (-22.7903, 106.7367) (-22.7943, 106.745) (-22.7985, 106.7533) (-22.8028, 106.7615) (-22.8071, 106.7699) (-22.8115, 106.7782) (-22.816, 106.7865) (-22.8206, 106.795) (-22.8253, 106.8034) (-22.83, 106.8118) (-22.8348, 106.8204) (-22.8397, 106.8289) (-22.8447, 106.8374) (-22.8498, 106.8461) (-22.855, 106.8547) (-22.8602, 106.8633) (-22.8834, 106.9019) (-22.9063, 106.9406) (-22.9286, 106.9797) (-22.9455, 107.0093) (-22.962, 107.039) (-22.9784, 107.0689) (-22.9965, 107.1022) (-23.0144, 107.1356) (-23.032, 107.1692) (-23.0514, 107.2063) (-23.0705, 107.2435) (-23.0892, 107.2809) (-23.1097, 107.3218) (-23.1298, 107.3628) (-23.1496, 107.404) (-23.171, 107.4487) (-23.192, 107.4937) (-23.2127, 107.5388) (-23.2349, 107.5874) (-23.2567, 107.6362) (-23.2781, 107.6852) (-23.301, 107.7378) (-23.3235, 107.7906) (-23.3455, 107.8436) (-23.369, 107.9001) (-23.392, 107.9569) (-23.4144, 108.0139) (-23.4383, 108.0745) (-23.4617, 108.1353) (-23.4845, 108.1963) (-23.5087, 108.261) (-23.5323, 108.3258) (-23.5553, 108.3909) (-23.5797, 108.4596) (-23.6034, 108.5286) (-23.6265, 108.5977) (-23.6692, 108.7256) (-23.7099, 108.8542) (-23.7487, 108.9834) knots 0 0 0 0 0.057795 0.057795 0.057795 0.089038 0.089038 0.089038 0.118617 0.118617 0.118617 0.14653 0.14653 0.14653 0.172778 0.172778 0.172778 0.19736 0.19736 0.19736 0.220277 0.220277 0.220277 0.241529 0.241529 0.241529 0.261115 0.261115 0.261115 0.279036 0.279036 0.279036 0.295292 0.295292 0.295292 0.309882 0.309882 0.309882 0.329164 0.329164 0.329164 0.333477 0.333477 0.333477 0.337694 0.337694 0.337694 0.34182 0.34182 0.34182 0.345864 0.345864 0.345864 0.349834 0.349834 0.349834 0.353742 0.353742 0.353742 0.3576 0.3576 0.3576 0.361424 0.361424 0.361424 0.365232 0.365232 0.365232 0.369048 0.369048 0.369048 0.372899 0.372899 0.372899 0.376819 0.376819 0.376819 0.380853 0.380853 0.380853 0.385052 0.385052 0.385052 0.389482 0.389482 0.389482 0.394225 0.394225 0.394225 0.399381 0.399381 0.399381 0.405067 0.405067 0.405067 0.411413 0.411413 0.411413 0.418548 0.418548 0.418548 0.426565 0.426565 0.426565 0.435472 0.435472 0.435472 0.445133 0.445133 0.445133 0.45436 0.45436 0.45436 0.5 0.5 0.5 0.54564 0.54564 0.54564 0.554867 0.554867 0.554867 0.564528 0.564528 0.564528 0.573435 0.573435 0.573435 0.581452 0.581452 0.581452 0.588587 0.588587 0.588587 0.594933 0.594933 0.594933 0.600619 0.600619 0.600619 0.605775 0.605775 0.605775 0.610518 0.610518 0.610518 0.614948 0.614948 0.614948 0.619147 0.619147 0.619147 0.623181 0.623181 0.623181 0.627101 0.627101 0.627101 0.630952 0.630952 0.630952 0.634768 0.634768 0.634768 0.638576 0.638576 0.638576 0.6424 0.6424 0.6424 0.646258 0.646258 0.646258 0.650166 0.650166 0.650166 0.654136 0.654136 0.654136 0.65818 0.65818 0.65818 0.662306 0.662306 0.662306 0.666523 0.666523 0.666523 0.670836 0.670836 0.670836 0.690118 0.690118 0.690118 0.704708 0.704708 0.704708 0.720964 0.720964 0.720964 0.738885 0.738885 0.738885 0.758471 0.758471 0.758471 0.779723 0.779723 0.779723 0.80264 0.80264 0.80264 0.827222 0.827222 0.827222 0.85347 0.85347 0.85347 0.881383 0.881383 0.881383 0.910962 0.910962 0.910962 0.942205 0.942205 0.942205 1 1 1 1
  arc A218 (-26.0399, 107.1057) -> (-26.8972, 106.3246) centre (0.0435, 77.6158) ccw
  spline S17 degree 3 poles (-28.9795, 104.2177) (-28.8545, 104.1671) (-28.7302, 104.1146) (-28.6069, 104.0602) (-28.5401, 104.0307) (-28.4737, 104.0007) (-28.4075, 103.9701) (-28.3449, 103.9412) (-28.2825, 103.9116) (-28.2204, 103.8816) (-28.1617, 103.8532) (-28.1034, 103.8243) (-28.0453, 103.7948) (-27.9906, 103.7672) (-27.9362, 103.739) (-27.8821, 103.7104) (-27.8314, 103.6836) (-27.7809, 103.6563) (-27.7307, 103.6286) (-27.6838, 103.6027) (-27.6372, 103.5765) (-27.5909, 103.5498) (-27.5479, 103.5251) (-27.5051, 103.5) (-27.4626, 103.4745) (-27.4234, 103.451) (-27.3844, 103.4272) (-27.3456, 103.403) (-27.3101, 103.3808) (-27.2748, 103.3584) (-27.2397, 103.3356) (-27.2079, 103.315) (-27.1763, 103.2941) (-27.1448, 103.2729) (-27.1166, 103.2539) (-27.0885, 103.2346) (-27.0606, 103.215) (-27.0238, 103.1892) (-26.9873, 103.1628) (-26.9511, 103.1362) (-26.943, 103.1302) (-26.9349, 103.1242) (-26.9267, 103.1183) (-26.9188, 103.1126) (-26.9107, 103.1069) (-26.9026, 103.1013) (-26.8947, 103.0958) (-26.8868, 103.0904) (-26.8788, 103.085) (-26.8709, 103.0798) (-26.863, 103.0746) (-26.8551, 103.0695) (-26.8473, 103.0645) (-26.8394, 103.0596) (-26.8315, 103.0548) (-26.8238, 103.05) (-26.8159, 103.0453) (-26.8081, 103.0407) (-26.8003, 103.0362) (-26.7925, 103.0317) (-26.7846, 103.0274) (-26.7768, 103.0231) (-26.7689, 103.0188) (-26.761, 103.0147) (-26.7531, 103.0106) (-26.7452, 103.0066) (-26.7372, 103.0027) (-26.7292, 102.9989) (-26.7211, 102.9951) (-26.713, 102.9914) (-26.7048, 102.9878) (-26.6965, 102.9842) (-26.6882, 102.9808) (-26.6797, 102.9773) (-26.6712, 102.974) (-26.6626, 102.9709) (-26.6538, 102.9676) (-26.6449, 102.9646) (-26.6359, 102.9617) (-26.6266, 102.9587) (-26.6172, 102.9559) (-26.6077, 102.9534) (-26.5977, 102.9507) (-26.5877, 102.9482) (-26.5776, 102.9461) (-26.5667, 102.9438) (-26.5558, 102.9418) (-26.5449, 102.9401) (-26.533, 102.9383) (-26.521, 102.9369) (-26.509, 102.9359) (-26.4958, 102.9349) (-26.4825, 102.9344) (-26.4693, 102.9344) (-26.4545, 102.9344) (-26.4396, 102.9351) (-26.4249, 102.9366) (-26.4083, 102.9382) (-26.3918, 102.9407) (-26.3755, 102.9442) (-26.3572, 102.9481) (-26.3391, 102.9531) (-26.3215, 102.9593) (-26.3019, 102.9662) (-26.2828, 102.9745) (-26.2643, 102.9842) (-26.2443, 102.9947) (-26.2251, 103.0067) (-26.2072, 103.0204) (-26.1901, 103.0335) (-26.1741, 103.048) (-26.1584, 103.0628) (-26.0808, 103.1359) (-26.0097, 103.2153) (-25.9348, 103.291) (-25.86, 103.3667) (-25.7814, 103.4388) (-25.7092, 103.5173) (-25.6947, 103.5331) (-25.6803, 103.5492) (-25.6675, 103.5665) (-25.654, 103.5846) (-25.6422, 103.6039) (-25.6319, 103.6241) (-25.6225, 103.6426) (-25.6144, 103.6618) (-25.6077, 103.6815) (-25.6017, 103.6992) (-25.5969, 103.7174) (-25.5932, 103.7357) (-25.5899, 103.7521) (-25.5876, 103.7686) (-25.5862, 103.7852) (-25.5849, 103.7999) (-25.5844, 103.8148) (-25.5845, 103.8296) (-25.5847, 103.8429) (-25.5853, 103.8561) (-25.5866, 103.8693) (-25.5877, 103.8813) (-25.5892, 103.8933) (-25.5911, 103.9051) (-25.5929, 103.9161) (-25.595, 103.9269) (-25.5975, 103.9377) (-25.5998, 103.9478) (-25.6023, 103.9578) (-25.6051, 103.9678) (-25.6078, 103.9772) (-25.6107, 103.9866) (-25.6138, 103.9959) (-25.6168, 104.0048) (-25.6199, 104.0137) (-25.6233, 104.0225) (-25.6265, 104.031) (-25.6299, 104.0395) (-25.6335, 104.0479) (-25.637, 104.0562) (-25.6407, 104.0644) (-25.6444, 104.0726) (-25.6482, 104.0807) (-25.652, 104.0887) (-25.656, 104.0967) (-25.66, 104.1046) (-25.6641, 104.1125) (-25.6683, 104.1203) (-25.6725, 104.1282) (-25.6768, 104.136) (-25.6812, 104.1438) (-25.6856, 104.1516) (-25.6902, 104.1594) (-25.6948, 104.1671) (-25.6995, 104.1749) (-25.7043, 104.1827) (-25.7091, 104.1904) (-25.7141, 104.1982) (-25.7191, 104.206) (-25.7242, 104.2138) (-25.7294, 104.2217) (-25.7346, 104.2295) (-25.74, 104.2373) (-25.7454, 104.2452) (-25.7509, 104.2531) (-25.7565, 104.2609) (-25.7622, 104.269) (-25.768, 104.2769) (-25.7738, 104.2848) (-25.7798, 104.2929) (-25.7859, 104.301) (-25.792, 104.309) (-25.819, 104.3449) (-25.8458, 104.3811) (-25.8721, 104.4176) (-25.892, 104.4453) (-25.9116, 104.4731) (-25.9309, 104.5011) (-25.9525, 104.5323) (-25.9738, 104.5637) (-25.9948, 104.5953) (-26.018, 104.6301) (-26.0408, 104.6651) (-26.0634, 104.7004) (-26.088, 104.7389) (-26.1123, 104.7776) (-26.1362, 104.8165) (-26.1622, 104.8587) (-26.1878, 104.9012) (-26.2131, 104.9439) (-26.2403, 104.9899) (-26.2671, 105.0362) (-26.2935, 105.0827) (-26.3218, 105.1326) (-26.3496, 105.1828) (-26.377, 105.2332) (-26.4063, 105.287) (-26.4351, 105.341) (-26.4634, 105.3954) (-26.4935, 105.4531) (-26.5231, 105.5111) (-26.5522, 105.5694) (-26.583, 105.6312) (-26.6132, 105.6932) (-26.6429, 105.7555) (-26.6743, 105.8214) (-26.7051, 105.8874) (-26.7353, 105.9538) (-26.7912, 106.0765) (-26.8451, 106.2002) (-26.8972, 106.3246) knots 0 0 0 0 0.057795 0.057795 0.057795 0.089038 0.089038 0.089038 0.118617 0.118617 0.118617 0.14653 0.14653 0.14653 0.172778 0.172778 0.172778 0.19736 0.19736 0.19736 0.220277 0.220277 0.220277 0.241529 0.241529 0.241529 0.261115 0.261115 0.261115 0.279036 0.279036 0.279036 0.295292 0.295292 0.295292 0.309882 0.309882 0.309882 0.329164 0.329164 0.329164 0.333477 0.333477 0.333477 0.337694 0.337694 0.337694 0.34182 0.34182 0.34182 0.345864 0.345864 0.345864 0.349834 0.349834 0.349834 0.353742 0.353742 0.353742 0.3576 0.3576 0.3576 0.361424 0.361424 0.361424 0.365232 0.365232 0.365232 0.369048 0.369048 0.369048 0.372899 0.372899 0.372899 0.376819 0.376819 0.376819 0.380853 0.380853 0.380853 0.385052 0.385052 0.385052 0.389482 0.389482 0.389482 0.394225 0.394225 0.394225 0.399381 0.399381 0.399381 0.405067 0.405067 0.405067 0.411413 0.411413 0.411413 0.418548 0.418548 0.418548 0.426565 0.426565 0.426565 0.435472 0.435472 0.435472 0.445133 0.445133 0.445133 0.45436 0.45436 0.45436 0.5 0.5 0.5 0.54564 0.54564 0.54564 0.554867 0.554867 0.554867 0.564528 0.564528 0.564528 0.573435 0.573435 0.573435 0.581452 0.581452 0.581452 0.588587 0.588587 0.588587 0.594933 0.594933 0.594933 0.600619 0.600619 0.600619 0.605775 0.605775 0.605775 0.610518 0.610518 0.610518 0.614948 0.614948 0.614948 0.619147 0.619147 0.619147 0.623181 0.623181 0.623181 0.627101 0.627101 0.627101 0.630952 0.630952 0.630952 0.634768 0.634768 0.634768 0.638576 0.638576 0.638576 0.6424 0.6424 0.6424 0.646258 0.646258 0.646258 0.650166 0.650166 0.650166 0.654136 0.654136 0.654136 0.65818 0.65818 0.65818 0.662306 0.662306 0.662306 0.666523 0.666523 0.666523 0.670836 0.670836 0.670836 0.690118 0.690118 0.690118 0.704708 0.704708 0.704708 0.720964 0.720964 0.720964 0.738885 0.738885 0.738885 0.758471 0.758471 0.758471 0.779723 0.779723 0.779723 0.80264 0.80264 0.80264 0.827222 0.827222 0.827222 0.85347 0.85347 0.85347 0.881383 0.881383 0.881383 0.910962 0.910962 0.910962 0.942205 0.942205 0.942205 1 1 1 1
  arc A219 (-28.9795, 104.2177) -> (-29.7505, 103.3512) centre (0.0435, 77.6158) ccw